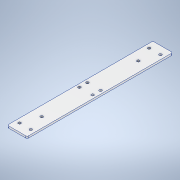
# Autodesk Inventor part: BedCarriageB
Saved by Autodesk Inventor 2020.2 (Build 242310000, 310)
## iProperties
Created: 2020-08-19
Part Number: BedCarriageB
Material: Generic
Document SubType Name: Modeling
Designer: JK
Density: 1 g/cm^3
Appearance: Aluminum - Flat
Author: JK
Autodesk Inventor part; units mm, degrees
ref_plane "YZ Plane" through (0, 0, 0) normal (1, 0, 0) x (0, 1, 0)
ref_plane "XZ Plane" through (0, 0, 0) normal (0, 1, 0) x (-1, 0, 0)
ref_plane "XY Plane" through (0, 0, 0) normal (0, 0, 1) x (1, 0, 0)
sketch "Sketch1" plane through (0, 0, 0) normal (0, 1, 0) x (-1, 0, 0)
  line L0 (-15, 110) -> (15, 110)
  line L1 (15, 110) -> (15, -110)
  line L2 (15, -110) -> (-15, -110)
  line L3 (-15, -110) -> (-15, 110)
  line L4 (-15, 110) -> (15, -110) construction
  line L5 (15, 110) -> (-15, -110) construction
  circle A0 centre (8.5, 98) radius 2
  circle A1 centre (-8.5, 98) radius 2
  circle A2 centre (8.5, -98) radius 2
  circle A3 centre (-8.5, -98) radius 2
  circle A4 centre (0, 73) radius 2
  circle A5 centre (0, -73) radius 2
  circle A6 centre (10, 6) radius 2
  circle A7 centre (10, -6) radius 2
  circle A8 centre (-10, 6) radius 2
  circle A9 centre (-10, -6) radius 2
  point P0 (0, 0)
  point P1 (0, 0)
  dimension "d0" = 30
  dimension "d1" = 220
  dimension "d2" = 17
  dimension "d3" = 4
  dimension "d4" = 25
  dimension "d5" = 12
  dimension "d7" = 12
  dimension "d8" = 25
  dimension "d9" = 4
  dimension "d10" = 12
  dimension "d11" = 20
  dimension "d12" = 6
  dimension "d13" = 10
  dimension "d14" = 8.5
  constraints: 12 end point, 10 centre point, 8 equal radius, 6 vertical alignment, 4 horizontal alignment, 3 midpoint, 2 parallel, 1 horizontal, 1 perpendicular
  measures "d0" distance of L1.end L2.end
  measures "d1" distance of L0.end L1.end
  measures "d2" distance of A2.centre A3.centre
  measures "d3" diameter of A2
  measures "d4" vertical distance of A2.centre A5.centre
  measures "d5" distance from line of L2 A2.centre
  measures "d7" distance from line of L0 A0.centre
  measures "d8" vertical distance of A0.centre A4.centre
  measures "d9" diameter of A7
  measures "d10" distance of A6.centre A7.centre
  measures "d11" distance of A7.centre A9.centre
  measures "d12" vertical distance of point (0, 0) A7.centre
  measures "d13" horizontal distance of point (0, 0) A9.centre
  measures "d14" horizontal distance of point (0, 0) A2.centre
extrude "Extrusion1" add sketch "Sketch1" along normal blind 3
fillet "Fillet1" radius 2 4 edges at (15, 1.5, 110) (15, 1.5, -110) (-15, 1.5, -110) (-15, 1.5, 110)
body "Solid1"
